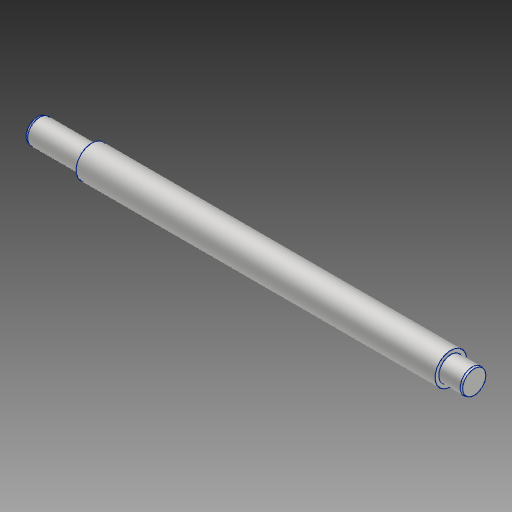
# Autodesk Inventor part: Dribblingwelle
Saved by Autodesk Inventor 2019.4 (Build 234330000, 330)
## iProperties
Part Number: Dribblingwelle
Material: Aluminium 6061
Document SubType Name: Modeling
Designer: rYan
Density: 2.7 g/cm^3
Appearance: Aluminium - flach
Mass: 7.44424 g
Surface Area: 18.1797 cm^2
Volume: 2.75712 cm^3
Author: rYan
Autodesk Inventor part; units mm, degrees
ref_plane "YZ Plane" through (0, 0, 0) normal (1, 0, 0) x (0, 1, 0)
ref_plane "XZ Plane" through (0, 0, 0) normal (0, 1, 0) x (-1, 0, 0)
ref_plane "XY Plane" through (0, 0, 0) normal (0, 0, 1) x (1, 0, 0)
sketch "Skizze1" plane through (0, 0, 0) normal (0, 0, 1) x (1, 0, 0)
  line L0 (-44.8, 0) -> (44.8, 0)
  line L1 (44.8, 0) -> (44.8, 2.5)
  line L2 (44.8, 2.5) -> (40, 2.5)
  line L3 (40, 2.5) -> (40, 3.25)
  line L4 (40, 3.25) -> (-33.7, 3.25)
  line L5 (-33.7, 3.25) -> (-33.7, 2.5)
  line L6 (-33.7, 2.5) -> (-44.8, 2.5)
  line L7 (-44.8, 2.5) -> (-44.8, 0)
  line L8 (0, 3.9) -> (0, -0.65) projected
  line L9 (-39.8, 2.5) -> (-39.8, 0) construction
  point P0 (0, 0)
  dimension "d1" = 4.8
  dimension "d2" = 5
  dimension "d4" = 6.5
  dimension "d18" = 5
  dimension "d20" = 79.8
  dimension "d22" = 6.1
  dimension "d23" = 5
  constraints: 18 end point, 7 perpendicular, 2 point on line, 1 horizontal, 1 midpoint, 1 other
  measures "d1" distance of L1.end L2.end
  measures "d2" diameter of L2 L0
  measures "d4" diameter of L4 L0
  measures "d18" diameter of L6 L0
  measures "d20" distance between parallel lines of L3 L9
  measures "d22" distance between parallel lines of L5 L9
  measures "d23" distance between parallel lines of L7 L9
revolve "Umdrehung1" add sketch "Skizze1" angle 360 about axis through (-44.8, 0, 0) along (1, 0, 0)
chamfer "Fase2" distance 0.4 angle 15 1 edges at (-44.8, -2.5, 0) measured on face at (-41.1, 2.4919, -0.2012)
chamfer "Fase3" distance 0.4 angle 15 1 edges at (44.8, -2.5, 0) measured on face at (41.6, 2.4919, -0.2012)
